Autodesk Inventor part; units mm, degrees
(part 2 of 2)
  spline S188 degree 2 poles (31.5955, -208.3531) (31.6548, -208.5112) (31.8746, -208.6816) (32.0524, -208.6816) knots 0 0 0 1 2 2 2
  spline S189 degree 2 poles (32.0524, -208.6816) (32.2204, -208.6816) (32.4402, -208.5211) (32.502, -208.3605) knots 0 0 0 1 2 2 2
  line L137 (35.2956, -208.9558) -> (33.4159, -208.9558)
  line L138 (33.4159, -208.9558) -> (33.4159, -208.5236)
  spline S190 degree 2 poles (33.4159, -208.5236) (33.6184, -208.3334) (33.9791, -207.9802) (34.152, -207.79) knots 0 0 0 1 2 2 2
  spline S191 degree 2 poles (34.152, -207.79) (34.5002, -207.4071) (34.7546, -206.9477) (34.7546, -206.7032) knots 0 0 0 1 2 2 2
  spline S192 degree 2 poles (34.7546, -206.7032) (34.7546, -206.5747) (34.6756, -206.3821) (34.604, -206.3203) knots 0 0 0 1 2 2 2
  spline S193 degree 2 poles (34.604, -206.3203) (34.5323, -206.2586) (34.3446, -206.1968) (34.231, -206.1968) knots 0 0 0 1 2 2 2
  spline S194 degree 2 poles (34.231, -206.1968) (34.1223, -206.1968) (33.9, -206.2512) (33.7987, -206.2931) knots 0 0 0 1 2 2 2
  spline S195 degree 2 poles (33.7987, -206.2931) (33.7123, -206.3277) (33.5517, -206.4265) (33.5023, -206.4611) knots 0 0 0 1 2 2 2
  line L139 (33.5023, -206.4611) -> (33.4801, -206.4611)
  line L140 (33.4801, -206.4611) -> (33.4801, -206.0264)
  spline S196 degree 2 poles (33.4801, -206.0264) (33.6061, -205.9646) (34.0581, -205.8436) (34.2606, -205.8436) knots 0 0 0 1 2 2 2
  spline S197 degree 2 poles (34.2606, -205.8436) (34.6879, -205.8436) (35.1696, -206.2956) (35.1696, -206.6809) knots 0 0 0 1 2 2 2
  spline S198 degree 2 poles (35.1696, -206.6809) (35.1696, -206.8612) (35.0856, -207.1626) (35.0115, -207.291) knots 0 0 0 1 2 2 2
  spline S199 degree 2 poles (35.0115, -207.291) (34.9374, -207.4244) (34.7225, -207.6862) (34.604, -207.8122) knots 0 0 0 1 2 2 2
  spline S200 degree 2 poles (34.604, -207.8122) (34.4113, -208.0222) (33.9395, -208.4717) (33.7987, -208.6026) knots 0 0 0 1 2 2 2
  line L141 (33.7987, -208.6026) -> (35.2956, -208.6026)
  line L142 (35.2956, -208.6026) -> (35.2956, -208.9558)
  spline S201 degree 2 poles (37.6297, -207.9678) (37.6297, -208.2025) (37.4741, -208.6001) (37.3432, -208.7335) knots 0 0 0 1 2 2 2
  spline S202 degree 2 poles (37.3432, -208.7335) (37.2074, -208.8743) (36.8665, -209.02) (36.6615, -209.02) knots 0 0 0 1 2 2 2
  spline S203 degree 2 poles (36.6615, -209.02) (36.4565, -209.02) (36.1181, -208.8817) (35.9896, -208.7434) knots 0 0 0 1 2 2 2
  spline S204 degree 2 poles (35.9896, -208.7434) (35.8316, -208.5779) (35.6537, -208.0222) (35.6537, -207.6171) knots 0 0 0 1 2 2 2
  spline S205 degree 2 poles (35.6537, -207.6171) (35.6537, -207.2194) (35.8167, -206.5797) (35.9872, -206.3425) knots 0 0 0 1 2 2 2
  spline S206 degree 2 poles (35.9872, -206.3425) (36.1527, -206.1104) (36.6763, -205.851) (37.0196, -205.851) knots 0 0 0 1 2 2 2
  spline S207 degree 2 poles (37.0196, -205.851) (37.1209, -205.851) (37.2988, -205.8708) (37.3654, -205.893) knots 0 0 0 1 2 2 2
  line L143 (37.3654, -205.893) -> (37.3654, -206.2857)
  line L144 (37.3654, -206.2857) -> (37.3482, -206.2857)
  spline S208 degree 2 poles (37.3482, -206.2857) (37.2913, -206.2561) (37.0839, -206.2042) (36.9653, -206.2042) knots 0 0 0 1 2 2 2
  spline S209 degree 2 poles (36.9653, -206.2042) (36.5849, -206.2042) (36.1181, -206.718) (36.0736, -207.2219) knots 0 0 0 1 2 2 2
  spline S210 degree 2 poles (36.0736, -207.2219) (36.2194, -207.1206) (36.5256, -207.0094) (36.7084, -207.0094) knots 0 0 0 1 2 2 2
  spline S211 degree 2 poles (36.7084, -207.0094) (36.8863, -207.0094) (37.153, -207.0811) (37.2988, -207.1898) knots 0 0 0 1 2 2 2
  spline S212 degree 2 poles (37.2988, -207.1898) (37.4667, -207.3157) (37.6297, -207.706) (37.6297, -207.9678) knots 0 0 0 1 2 2 2
  spline S213 degree 2 poles (37.2148, -207.9851) (37.2148, -207.7974) (37.116, -207.543) (37.0073, -207.454) knots 0 0 0 1 2 2 2
  spline S214 degree 2 poles (37.0073, -207.454) (36.9258, -207.3898) (36.7232, -207.3478) (36.617, -207.3478) knots 0 0 0 1 2 2 2
  spline S215 degree 2 poles (36.617, -207.3478) (36.4738, -207.3478) (36.2045, -207.4343) (36.0736, -207.5158) knots 0 0 0 1 2 2 2
  spline S216 degree 2 poles (36.0736, -207.5158) (36.0712, -207.5603) (36.0662, -207.6442) (36.0662, -207.7085) knots 0 0 0 1 2 2 2
  spline S217 degree 2 poles (36.0662, -207.7085) (36.0662, -208.0246) (36.1897, -208.4124) (36.2836, -208.5137) knots 0 0 0 1 2 2 2
  spline S218 degree 2 poles (36.2836, -208.5137) (36.37, -208.61) (36.5578, -208.6866) (36.664, -208.6866) knots 0 0 0 1 2 2 2
  spline S219 degree 2 poles (36.664, -208.6866) (36.911, -208.6866) (37.2148, -208.3358) (37.2148, -207.9851) knots 0 0 0 1 2 2 2
  point P0 (0, 0)
  constraints: 2 other
emboss "Emboss1" sketch "Sketch14" operation cut depth 2.54 direction (-1, 0, 0)
sketch "Sketch16" plane through (5.08, 0, 0) normal (1, 0, 0) x (0, 0, -1)
  line L0 (-41.7074, -74.9522) -> (39.5726, -74.9522)
  line L1 (39.5726, -74.9522) -> (39.5726, -78.7622)
  line L2 (39.5726, -78.7622) -> (-41.7074, -78.7622)
  line L3 (-41.7074, -78.7622) -> (-41.7074, -74.9522)
  line L4 (22.7938, -210.0802) -> (-43.6417, -210.0802) projected
  point P0 (0, 0)
  point P1 (-43.6417, -212.6202)
  dimension "d193" = 135.128
  dimension "d195" = 3.81
  constraints: 8 end point, 2 parallel, 1 horizontal, 1 perpendicular
  measures "d193" distance between parallel lines of L4 L0
  measures "d195" distance between parallel lines of L0 L2
extrude "Extrusion13" add sketch "Sketch16" along normal blind 5.08
sketch "Sketch17" plane through (20.32, 33.2264, 20.9087) normal (0, 1, 0) x (1, 0, 0)
  line L0 (-4.318, 35.56) -> (0, 35.56) projected
  line L1 (-0.0061, 35.56) -> (0.0392, 35.56)
  line L2 (0, 64.9986) -> (0, -27.9146) projected
  line L3 (0, 35.5801) -> (0, 35.5243)
  line L4 (5, -24.7396) -> (5, 61.8236) projected
  line L5 (0, 35.56) -> (5, 35.56)
  line L6 (5, 35.56) -> (5, -0.0031)
  line L7 (5, -0.0031) -> (0, -0.0031)
  line L8 (0, -0.0031) -> (0, 35.56)
  point P0 (-20.32, 20.9087)
  point P1 (5, -23.8506)
  point P2 (5, 69.0626)
  point P3 (0.0392, 35.56)
  constraints: 12 end point, 4 point on line, 2 horizontal, 2 parallel, 1 perpendicular
extrude "Extrusion14" cut sketch "Sketch17" against normal blind 2.0066
sketch "Sketch18" plane through (0, 0, 0) normal (-1, 0, 0) x (0, 0, 1)
  arc A0 (46.6025, 33.0796) -> (48.6765, 31.0055) centre (48.5947, 32.9978) ccw projected
  circle A1 centre (48.5947, 32.9978) radius 4.5085
  arc A2 (-41.8691, 33.0796) -> (-43.9431, 31.0055) centre (-43.8613, 32.9978) ccw projected
  circle A3 centre (-43.8613, 32.9978) radius 4.5085
  arc A4 (-43.9431, -212.406) -> (-41.8691, -214.4801) centre (-43.8613, -214.3982) ccw projected
  circle A5 centre (-43.8613, -214.3982) radius 4.5085
  arc A6 (46.6025, -214.4801) -> (48.6765, -212.406) centre (48.5947, -214.3982) ccw projected
  circle A7 centre (48.5947, -214.3982) radius 4.5085
  point P0 (0, 0)
  dimension "d209" = 9.017
  dimension "d210" = 9.017
  dimension "d211" = 9.017
  dimension "d212" = 9.017
  constraints: 4 centre point, 4 coincident
  measures "d209" diameter of A1
  measures "d210" diameter of A3
  measures "d211" diameter of A5
  measures "d212" diameter of A7
extrude "Extrusion15" cut sketch "Sketch18" against normal blind 5
body "Solid1"
